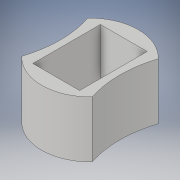
# Autodesk Inventor part: joint3_2part
Saved by Autodesk Inventor 2019 (Build 230136000, 136)
## iProperties
Created: 2019-12-29
Part Number: joint3_2part
Material: Типовые
Document SubType Name: Modeling
Designer: Петров Иван
Density: 1 g/cm^3
Appearance: По умолчанию
Author: Петров Иван
Autodesk Inventor part; units mm, degrees
ref_plane "YZ Plane" through (0, 0, 0) normal (1, 0, 0) x (0, 1, 0)
ref_plane "XZ Plane" through (0, 0, 0) normal (0, 1, 0) x (-1, 0, 0)
ref_plane "XY Plane" through (0, 0, 0) normal (0, 0, 1) x (1, 0, 0)
sketch "Эскиз1" plane through (0, 0, 0) normal (0, 1, 0) x (-1, 0, 0)
  arc A0 (-21.8781, -20.5267) -> (-21.8781, 20.5267) centre (-85.5896, 0) ccw
  arc A1 (21.8781, 20.5267) -> (-21.8781, 20.5267) centre (0, 0) ccw
  arc A2 (21.8781, 20.5267) -> (21.8781, -20.5267) centre (85.5896, 0) ccw
  arc A3 (-21.8781, -20.5267) -> (21.8781, -20.5267) centre (0, 0) ccw
  arc A4 (25.4245, 11.0214) -> (14.3699, 31.9141) centre (6.4664, 14.3613) ccw
  arc A5 (14.3699, 31.9141) -> (-14.3699, 31.9141) centre (0, 0) ccw
  arc A6 (-14.3699, 31.9141) -> (-25.4245, 11.0214) centre (-6.4664, 14.3613) ccw
  arc A7 (-25.8326, -10.0276) -> (-25.4245, 11.0214) centre (-79.2616, 1.5368) ccw
  arc A8 (-25.8326, -10.0276) -> (-15.5961, -31.3331) centre (-7.0183, -14.0999) ccw
  arc A9 (-15.5961, -31.3331) -> (15.5961, -31.3331) centre (0, 0) ccw
  arc A10 (15.5961, -31.3331) -> (25.8326, -10.0276) centre (7.0183, -14.0999) ccw
  arc A11 (25.4245, 11.0214) -> (25.8326, -10.0276) centre (79.2616, 1.5368) ccw
  line L0 (19.5667, 11.0214) -> (14.5667, 11.0214)
  line L1 (19.5667, -11.0214) -> (14.5667, -11.0214)
  line L2 (14.5667, -11.0214) -> (14.5667, 11.0214)
  line L3 (0, 0) -> (0, -4.3757)
  line L4 (-19.5667, 11.0214) -> (-14.5667, 11.0214)
  line L5 (-19.5667, -11.0214) -> (-14.5667, -11.0214)
  line L6 (-14.5667, -11.0214) -> (-14.5667, 11.0214)
  line L7 (14.5667, 11.0214) -> (14.5667, 21.0214)
  line L8 (14.5667, 21.0214) -> (-14.5667, 21.0214)
  line L9 (-14.5667, 21.0214) -> (-14.5667, 11.0214)
  line L10 (0, 0) -> (2.4849, 0)
  line L11 (14.5667, -11.0214) -> (14.5667, -21.0214)
  line L12 (14.5667, -21.0214) -> (-14.5667, -21.0214)
  line L13 (-14.5667, -21.0214) -> (-14.5667, -11.0214)
  point P0 (6.4664, -14.3613)
  point P1 (-6.4664, -14.3613)
  dimension "d0" = 5
  dimension "d1" = 5
  dimension "d2" = 10
  constraints: 28 end point, 26 point on circle, 12 centre point, 8 symmetric about line, 3 horizontal, 3 perpendicular, 2 vertical
  measures "d0" distance of L0.start L0.end
  measures "d1" distance of L1.start L1.end
  measures "d2" distance of L0.end L7.end
extrude "Выдавливание1" add sketch "Эскиз1" along normal blind 35 contours A0 L5 L13 L12 L11 L1 A2 A3 | A0 L4 L6 L5 | A0 A1 A2 L0 L7 L8 L9 L4 | L1 L2 L0 A2
